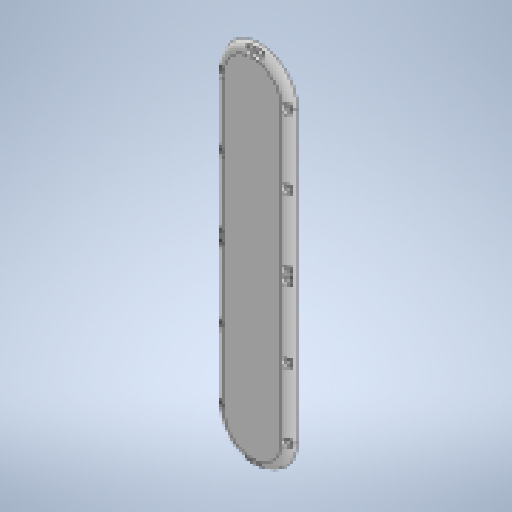
# Autodesk Inventor part: Merged J1 Side Logo Plates
Saved by Autodesk Inventor 2024 (Build 280153000, 153)
## iProperties
Created: 2023-08-31
Part Number: Merged J1 Side Logo Plates
Material: Generic
Document SubType Name: Modeling
Designer: byrne
Density: 1 g/cm^3
Appearance: Default
Author: byrne
Autodesk Inventor part; units mm, degrees
ref_plane "YZ Plane" through (0, 0, 0) normal (1, 0, 0) x (0, 1, 0)
ref_plane "XZ Plane" through (0, 0, 0) normal (0, 1, 0) x (-1, 0, 0)
ref_plane "XY Plane" through (0, 0, 0) normal (0, 0, 1) x (1, 0, 0)
sketch "Sketch1" plane through (0, 0, 0) normal (0, 0, 1) x (1, 0, 0)
  arc A0 (30, 230.9775) -> (-30, 230.9775) centre (0, 230.9775) ccw projected
  line L0 (30, 132.8093) -> (30, 230.9775) projected
  line L1 (30, 0) -> (30, 132.8093) projected
  arc A1 (-30, 0) -> (30, 0) centre (0, 0) ccw projected
  line L2 (-30, 98.1683) -> (-30, 0) projected
  line L3 (-30, 230.9775) -> (-30, 98.1683) projected
  circle A2 centre (-26.75, 118.8888) radius 1.7 projected
  circle A3 centre (-26.75, 112.0888) radius 1.7 projected
  circle A4 centre (-26.75, 175.4888) radius 1.7 projected
  circle A5 centre (-26.75, 230.9775) radius 1.7 projected
  circle A6 centre (-3.3, 257.5232) radius 1.7 projected
  circle A7 centre (3.3, 257.5232) radius 1.7 projected
  circle A8 centre (26.75, 230.9775) radius 1.7 projected
  circle A9 centre (26.75, 175.4888) radius 1.7 projected
  circle A10 centre (26.75, 118.8888) radius 1.7 projected
  circle A11 centre (26.75, 112.0888) radius 1.7 projected
  circle A12 centre (26.75, 55.4888) radius 1.7 projected
  circle A13 centre (26.75, 0) radius 1.7 projected
  circle A14 centre (3.3, -26.5457) radius 1.7 projected
  circle A15 centre (-3.3, -26.5457) radius 1.7 projected
  circle A16 centre (-26.75, 0) radius 1.7 projected
  circle A17 centre (-26.75, 55.4888) radius 1.7 projected
  point P0 (0, 0)
extrude "Extrusion1" add sketch "Sketch1" along normal blind 6
fillet "Fillet1" radius 7 4 edges at (-30, 49.0841, 6) (0, -30, 6) (30, 181.8934, 6) (0, 260.9775, 6)
sketch "Sketch2" plane through (0, 0, 6) normal (0, 0, 1) x (1, 0, 0)
  line L0 (-30, 230.9775) -> (-30, 0) projected
  arc A0 (-30, 0) -> (30, 0) centre (0, 0) ccw projected
  line L1 (30, 0) -> (30, 230.9775) projected
  arc A1 (30, 230.9775) -> (-30, 230.9775) centre (0, 230.9775) ccw projected
  circle A2 centre (-26.75, 55.4888) radius 1.7 projected
  circle A3 centre (26.75, 55.4888) radius 1.7 projected
  circle A4 centre (26.75, 112.0888) radius 1.7 projected
  circle A5 centre (26.75, 118.8888) radius 1.7 projected
  circle A6 centre (26.75, 175.4888) radius 1.7 projected
  circle A7 centre (-26.75, 175.4888) radius 1.7 projected
  circle A8 centre (-26.75, 112.0888) radius 1.7 projected
  circle A9 centre (-26.75, 118.8888) radius 1.7 projected
  circle A10 centre (-26.75, 0) radius 1.7 projected
  circle A11 centre (-3.3, -26.5457) radius 1.7 projected
  circle A12 centre (3.3, -26.5457) radius 1.7 projected
  circle A13 centre (26.75, 0) radius 1.7 projected
  circle A14 centre (26.75, 230.9775) radius 1.7 projected
  circle A15 centre (3.3, 257.5232) radius 1.7 projected
  circle A16 centre (-3.3, 257.5232) radius 1.7 projected
  circle A17 centre (-26.75, 230.9775) radius 1.7 projected
  circle A18 centre (-3.3, -26.5457) radius 3.7
  circle A19 centre (3.3, -26.5457) radius 3.7
  circle A20 centre (-26.75, 0) radius 3.7
  circle A21 centre (26.75, 0) radius 3.7
  circle A22 centre (-26.75, 55.4888) radius 3.7
  circle A23 centre (26.75, 55.4888) radius 3.7
  circle A24 centre (26.75, 112.0888) radius 3.7
  circle A25 centre (26.75, 118.8888) radius 3.7
  circle A26 centre (-26.75, 118.8888) radius 3.7
  circle A27 centre (-26.75, 112.0888) radius 3.7
  circle A28 centre (-26.75, 175.4888) radius 3.7
  circle A29 centre (26.75, 175.4888) radius 3.7
  circle A30 centre (-26.75, 230.9775) radius 3.7
  circle A31 centre (26.75, 230.9775) radius 3.7
  circle A32 centre (3.3, 257.5232) radius 3.7
  circle A33 centre (-3.3, 257.5232) radius 3.7
  point P0 (0, 0)
  point P1 (0, 259.1965)
  point P2 (0, 255.8499)
  point P3 (25.2905, 115.4888)
  point P4 (28.2095, 115.4888)
  point P5 (-25.2905, 115.4888)
  point P6 (-28.2095, 115.4888)
  point P7 (0, -24.8723)
  point P8 (0, -28.219)
  dimension "d2" = 2
  dimension "d3" = 2
  dimension "d4" = 2
  dimension "d5" = 2
  dimension "d6" = 2
  dimension "d7" = 2
  dimension "d8" = 2
  dimension "d9" = 2
  dimension "d10" = 2
  dimension "d11" = 2
  dimension "d12" = 2
  dimension "d13" = 2
  dimension "d14" = 2
  dimension "d15" = 2
  dimension "d16" = 2
  dimension "d17" = 2
  constraints: 16 centre point
  measures "d2" radial gap between concentric circles of A11 A18
  measures "d3" radial gap between concentric circles of A12 A19
  measures "d4" radial gap between concentric circles of A10 A20
  measures "d5" radial gap between concentric circles of A13 A21
  measures "d6" radial gap between concentric circles of A2 A22
  measures "d7" radial gap between concentric circles of A3 A23
  measures "d8" radial gap between concentric circles of A4 A24
  measures "d9" radial gap between concentric circles of A5 A25
  measures "d10" radial gap between concentric circles of A9 A26
  measures "d11" radial gap between concentric circles of A8 A27
  measures "d12" radial gap between concentric circles of A7 A28
  measures "d13" radial gap between concentric circles of A6 A29
  measures "d14" radial gap between concentric circles of A17 A30
  measures "d15" radial gap between concentric circles of A14 A31
  measures "d16" radial gap between concentric circles of A15 A32
  measures "d17" radial gap between concentric circles of A16 A33
extrude "Extrusion2" cut sketch "Sketch2" against normal blind 3 contours A1 A30 L0 | L0 A30 A1 | A28 L0 | L0 A28 | A33 A1 | A1 A33 A32 | A33 A32 A1 | A32 A33 | A26 A27 L0 | L0 A26 | A32 A1 | A27 A26 L0 | L0 A27 | A27 A26 | A31 L1 A1 | A1 L1 A31 | A22 L0 | L0 A22 | A29 L1 | L1 A29 | A20 A0 L0 | L0 A0 A20 | A25 L1 | L1 A25 A24 | A25 A24 L1 | A24 A25 | A18 A19 A0 | A0 A18 | A24 L1 | A19 A0 A18 | A18 A19 | A23 L1 | L1 A23 | A0 A19 | A21 A0 L1 | L1 A0 A21 | A2 | A3 | A4 | A5 | A6 | A7 | A8 | A9 | A10 | A11 | A12 | A13 | A14 | A15 | A16 | A17 picked at (-0.9389, 256.0581) picked at (0.9158, 255.9618) picked at (-29.4833, 118.8888) picked at (-29.4833, 112.0888) picked at (29.4833, 118.8888) picked at (29.4833, 112.0888) picked at (-0.9389, -25.0806) picked at (0.9158, -24.9843)
body "Solid1"
